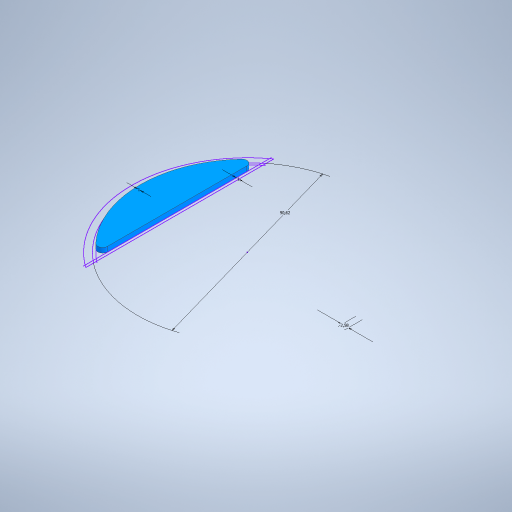
# Autodesk Inventor part: Test_PCB
Saved by Autodesk Inventor 2024 (Build 280153000, 153)
## iProperties
Created: 2025-01-20
Part Number: Test_PCB
Material: Générique
Document SubType Name: Modeling
Designer: malam
Density: 1 g/cm^3
Appearance: Par défaut
Author: malam
Autodesk Inventor part; units mm, degrees
ref_plane "YZ Plane" through (0, 0, 0) normal (1, 0, 0) x (0, 1, 0)
ref_plane "XZ Plane" through (0, 0, 0) normal (0, 1, 0) x (-1, 0, 0)
ref_plane "XY Plane" through (0, 0, 0) normal (0, 0, 1) x (1, 0, 0)
sketch "Esquisse1" plane through (0, 0, 0) normal (0, 1, 0) x (-1, 0, 0)
  arc A0 (28, -38.8517) -> (28, 38.8517) centre (0, 0) ccw
  arc A1 (28, -35.623) -> (28, 35.623) centre (0, 0) ccw
  line L0 (28, 32.55) -> (28, -32.55)
  line L1 (28, 32.55) -> (28, 38.8517)
  line L2 (28, -32.55) -> (28, -38.8517)
  arc A2 (27.382, -34.8368) -> (27.382, 34.8368) centre (0, 0) ccw
  line L3 (29, -38.8517) -> (29, 38.8517)
  point P0 (0, 0)
  point P1 (29, 33.5019)
  point P2 (29, -33.5019)
  dimension "d0" = 90.62
  dimension "d1" = 2.58
  dimension "d2" = 1
  dimension "d3" = 1
  constraints: 8 end point, 6 point on circle, 3 centre point, 3 point on line, 2 vertical
  measures "d0" diameter of A1
  measures "d1" radial gap between concentric circles of A1 A0
  measures "d2" radial gap between concentric circles of A1 A2
  measures "d3" distance between parallel lines of L0 L3
extrude "Extrusion1" add sketch "Esquisse1" along normal blind 2 contours L3 A2
fillet "Congé1" radius 2 2 edges at (-29, 1, 33.5019) (-29, 1, -33.5019)
